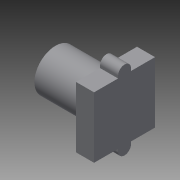
# Autodesk Inventor part: camera_Fatshark_600TVL
Saved by Autodesk Inventor 2015 SP1 (Build 190203100, 203)
## iProperties
Created: 2015-09-01
Part Number: camera_Fatshark_600TVL
Material: Generic
Document SubType Name: Modeling
Designer: Alexandre Cherpillod
Density: 1 g/cm^3
Appearance: Default
Author: Alexandre Cherpillod
Autodesk Inventor part; units mm, degrees
ref_plane "YZ Plane" through (0, 0, 0) normal (1, 0, 0) x (0, 1, 0)
ref_plane "XZ Plane" through (0, 0, 0) normal (0, 1, 0) x (-1, 0, 0)
ref_plane "XY Plane" through (0, 0, 0) normal (0, 0, 1) x (1, 0, 0)
sketch "Sketch1" plane through (0, 0, 0) normal (1, 0, 0) x (0, 1, 0)
  circle A0 centre (0, 0) radius 7
  dimension "d0" = 14
  constraints: 1 centre point, 1 coincident
  measures "d0" diameter of A0
extrude "Extrusion1" add sketch "Sketch1" along normal blind 17
sketch "Sketch2" plane through (17, 0, 0) normal (1, 0, 0) x (0, 0, -1)
  line L0 (-10.15, -10.15) -> (10.15, -10.15)
  line L1 (10.15, -10.15) -> (10.15, 10.15)
  line L2 (10.15, 10.15) -> (-10.15, 10.15)
  line L3 (-10.15, 10.15) -> (-10.15, -10.15)
  line L4 (-10.15, -10.15) -> (10.15, 10.15) construction
  line L5 (10.15, -10.15) -> (-10.15, 10.15) construction
  point P0 (0, 0)
  dimension "d3" = 20.3
  dimension "d4" = 20.3
  constraints: 12 end point, 2 midpoint, 2 parallel, 1 horizontal, 1 perpendicular
  measures "d3" distance of L2.end L1.end
  measures "d4" distance of L0.end L1.end
extrude "Extrusion2" add sketch "Sketch2" along normal blind 6
sketch "Sketch3" plane through (23, 0, 0) normal (1, 0, 0) x (0, 0, -1)
  arc A0 (-10.95, 2.15) -> (-10.95, -2.15) centre (-10.95, 0) ccw
  arc A1 (10.95, -2.15) -> (10.95, 2.15) centre (10.95, 0) ccw
  line L0 (10.15, -10.15) -> (10.15, 10.15) projected
  line L1 (-10.15, 10.15) -> (-10.15, -10.15) projected
  line L2 (-10.95, 2.15) -> (-10.15, 2.15)
  line L3 (-10.95, -2.15) -> (-10.15, -2.15)
  line L4 (10.95, 2.15) -> (10.15, 2.15)
  line L5 (10.95, -2.15) -> (10.15, -2.15)
  line L6 (-10.15, 2.15) -> (-10.15, -2.15)
  line L7 (10.15, 2.15) -> (10.15, -2.15)
  point P0 (0, 0)
  dimension "d7" = 4.3
  dimension "d8" = 4.3
  dimension "d9" = 0.8
  dimension "d10" = 0.8
  constraints: 12 end point, 6 point on line, 4 perpendicular, 4 point on circle, 3 tangent, 2 centre point, 1 vertical
  measures "d7" diameter of A0
  measures "d8" diameter of A1
  measures "d9" distance from line of L0 A1.centre
  measures "d10" distance from line of L1 A0.centre
extrude "Extrusion3" add sketch "Sketch3" against normal up to surface (6 mm away)
body "Solid1"
